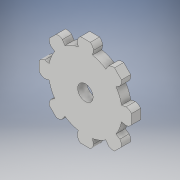
# Autodesk Inventor part: Servo Gear
Saved by Autodesk Inventor 2017 (Build 210142000, 142)
## iProperties
Created: 2018-03-04
Part Number: Servo Gear
Material: Generic
Document SubType Name: Modeling
Designer: Russ
Density: 1 g/cm^3
Appearance: Default
Author: Russ
Autodesk Inventor part; units mm, degrees
ref_plane "YZ Plane" through (0, 0, 0) normal (1, 0, 0) x (0, 1, 0)
ref_plane "XZ Plane" through (0, 0, 0) normal (0, 1, 0) x (-1, 0, 0)
ref_plane "XY Plane" through (0, 0, 0) normal (0, 0, 1) x (1, 0, 0)
sketch "Sketch1" plane through (0, 0, 0) normal (0, 0, 1) x (1, 0, 0)
  arc A0 (-2.0086, 7.3505) -> (2.0086, 7.3505) centre (0, 0) ccw
  line L0 (0, 7.62) -> (0, 9.525)
  line L1 (0, 9.525) -> (1.016, 9.525)
  line L2 (0, 9.525) -> (-1.016, 9.525)
  arc A1 (-1.4866, 7.4736) -> (1.4866, 7.4736) centre (0, 0) ccw
  line L3 (-1.4866, 7.4736) -> (-1.8582, 9.342)
  line L4 (-2.916, 7.04) -> (-3.6451, 8.8)
  line L5 (-4.2334, 6.3358) -> (-5.2918, 7.9197)
  line L6 (-5.3882, 5.3882) -> (-6.7352, 6.7352)
  line L7 (-6.3358, 4.2334) -> (-7.9197, 5.2918)
  line L8 (-7.04, 2.916) -> (-8.8, 3.6451)
  line L9 (-7.04, -2.916) -> (-8.8, -3.6451)
  line L10 (-6.3358, -4.2334) -> (-7.9197, -5.2918)
  line L11 (-5.3882, -5.3882) -> (-6.7352, -6.7352)
  line L12 (-4.2334, -6.3358) -> (-5.2918, -7.9197)
  line L13 (-2.916, -7.04) -> (-3.6451, -8.8)
  line L14 (-1.4866, -7.4736) -> (-1.8582, -9.342)
  line L15 (0, -7.62) -> (0, -9.525)
  line L16 (1.4866, -7.4736) -> (1.8582, -9.342)
  line L17 (2.916, -7.04) -> (3.6451, -8.8)
  line L18 (4.2334, -6.3358) -> (5.2918, -7.9197)
  line L19 (5.3882, -5.3882) -> (6.7352, -6.7352)
  line L20 (6.3358, -4.2334) -> (7.9197, -5.2918)
  line L21 (7.04, -2.916) -> (8.8, -3.6451)
  line L22 (7.4736, -1.4866) -> (9.342, -1.8582)
  line L23 (7.62, 0) -> (9.525, 0)
  line L24 (7.4736, 1.4866) -> (9.342, 1.8582)
  line L25 (7.04, 2.916) -> (8.8, 3.6451)
  line L26 (6.3358, 4.2334) -> (7.9197, 5.2918)
  line L27 (5.3882, 5.3882) -> (6.7352, 6.7352)
  line L28 (4.2334, 6.3358) -> (5.2918, 7.9197)
  line L29 (2.916, 7.04) -> (3.6451, 8.8)
  line L30 (1.4866, 7.4736) -> (1.8582, 9.342)
  arc A2 (-1.4866, 7.4736) -> (1.4866, 7.4736) centre (0, 0) ccw
  arc A3 (-1.016, 9.525) -> (-1.6724, 8.4079) centre (-0.1056, 8.2386) ccw
  arc A4 (1.6724, 8.4079) -> (1.016, 9.525) centre (0.1056, 8.2386) ccw
  circle A5 centre (0, 0) radius 7.62
  line L31 (-1.4866, 7.4736) -> (-1.6724, 8.4079)
  line L32 (-1.016, 9.525) -> (1.016, 9.525)
  line L33 (1.6724, 8.4079) -> (1.4866, 7.4736)
  arc A6 (-1.016, 9.525) -> (-1.6724, 8.4079) centre (-0.1056, 8.2386) ccw
  arc A7 (1.6724, 8.4079) -> (1.016, 9.525) centre (0.1056, 8.2386) ccw
  point P0 (-7.4736, 1.4866)
  point P1 (-7.62, 0)
  point P2 (-7.4736, -1.4866)
  dimension "d0" = 15.24
  dimension "d1" = 360
  dimension "d2" = 1.016
  dimension "d3" = 1.016
  dimension "d4" = 1.905
  constraints: 68 end point, 14 point on circle, 7 centre point, 5 symmetric about line, 4 coincident, 3 concentric, 2 collinear, 1 perpendicular, 1 point on line, 1 vertical, 4 other
  measures "d0" diameter of A0
  measures "d2" distance of L1.start L1.end
  measures "d3" distance of L1.start L2.end
  measures "d4" distance of L0.start L1.start
extrude "Extrusion1" add sketch "Sketch1" along normal blind 1.905
pattern_circular "Circular Pattern1" count 8 over 360 about axis through (0, 0, 0) along (0, 0, 1) of "Extrusion1"
sketch "Sketch2" plane through (0, 0, 1.905) normal (0, 0, 1) x (1, 0, 0)
  circle A0 centre (0, 0) radius 1.6
  dimension "d10" = 3.2
  constraints: 1 centre point, 1 coincident
  measures "d10" diameter of A0
extrude "Extrusion2" cut sketch "Sketch2" against normal up to next
body "Solid1"
